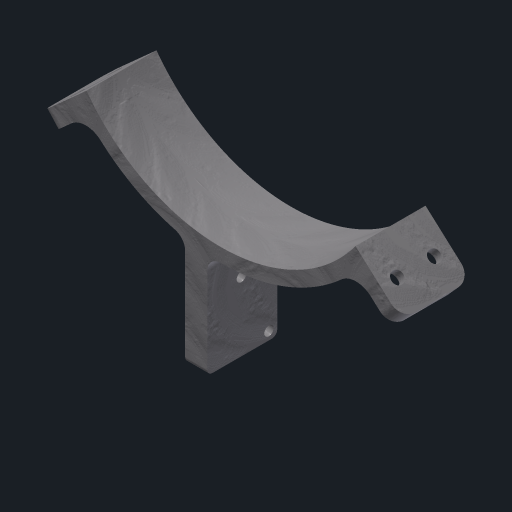
# Autodesk Inventor part: CANALETA_MOVIL
Saved by Autodesk Inventor 2024.3 (Build 283343000, 343)
## iProperties
Created: 2024-07-24
Part Number: CANALETA_MOVIL
Material: Steel, Mild, Welded
Document SubType Name: Modeling
Designer: Niler
Density: 7.85 g/cm^3
Appearance: Weld - Steel Mild
Author: Niler
Autodesk Inventor part; units mm, degrees
ref_plane "YZ Plane" through (0, 0, 0) normal (1, 0, 0) x (0, 1, 0)
ref_plane "XZ Plane" through (0, 0, 0) normal (0, 1, 0) x (-1, 0, 0)
ref_plane "XY Plane" through (0, 0, 0) normal (0, 0, 1) x (1, 0, 0)
sketch "Sketch1" plane through (0, 0, 0) normal (0, 0, 1) x (1, 0, 0)
  circle A0 centre (0, 0) radius 57.5
  circle A1 centre (0, 0) radius 60.5
  line L0 (0, 0) -> (-45, -40.4382)
  line L1 (0, 0) -> (0, 20.5864)
  line L2 (0, 0) -> (45, -40.4382)
  circle A2 centre (0, 0) radius 65.5
  line L3 (-45, -40.4382) -> (-48.719, -43.7802)
  line L4 (45, -40.4382) -> (48.719, -43.7802)
  line L5 (-4.7542, 3.7944) -> (-49.0104, -35.9754)
  line L6 (-49.0104, -35.9754) -> (-65.4381, -50.7378)
  line L7 (-48.719, -43.7802) -> (-61.4277, -55.2006)
  line L8 (-65.4381, -50.7378) -> (-61.4277, -55.2006)
  arc A3 (-43.6644, -48.8229) -> (-54.3446, -48.8356) centre (-48.9974, -54.786) ccw
  line L9 (49.0104, -35.9754) -> (65.4381, -50.7378)
  line L10 (48.719, -43.7802) -> (61.4277, -55.2006)
  line L11 (65.4381, -50.7378) -> (61.4277, -55.2006)
  arc A4 (54.3446, -48.8356) -> (43.6644, -48.8229) centre (48.9974, -54.786) ccw
  line L12 (4.7542, 3.7944) -> (49.0104, -35.9754)
  point P0 (45, -40.4382)
  point P1 (42.7686, -38.433)
  point P2 (-42.7686, -38.433)
  point P3 (-46.5455, -33.7604)
  point P4 (52.5246, -39.1333)
  point P5 (43.6644, -48.8229)
  point P6 (-48.7886, -35.7761)
  point P7 (48.7886, -35.7761)
  dimension "d0" = 115
  dimension "d1" = 3
  dimension "d2" = 90
  dimension "d5" = 5
  dimension "d6" = 6
  dimension "d7" = 25.4
  dimension "d8" = 8
  constraints: 28 end point, 8 symmetric about line, 7 point on circle, 4 collinear, 3 centre point, 3 point on line, 2 tangent, 1 coincident, 1 perpendicular, 1 vertical, 8 other
  measures "d2" distance of L2.end L0.end
  measures "d6" distance between parallel lines of L0 L5
  measures "d7" distance of L6.end point (-46.546, -33.76)
  measures "d8" radius of A3
extrude "Extrusion1" add sketch "Sketch1" along normal mid plane 25.4 contours A1 L3 A2 L6 L5 | L12 L9 A2 L4 A1 | A1 L4 A2 L3 | L7 L8 L6 A2 | A2 A3 L7 | L10 A4 A2 | A2 L9 L11 L10
fillet "Fillet1" radius 5 4 edges at (-63.4329, -52.9692, 12.7) (-63.4329, -52.9692, -12.7) (63.4329, -52.9692, 12.7) (63.4329, -52.9692, -12.7)
sketch "Sketch2" plane through (-54.3446, -48.8356, -12.7) normal (0.6684004, -0.7438017, 0) x (0.7438017, 0.6684004, 0)
  arc A0 (-9.5228, 5) -> (-4.5228, 0) centre (-4.5228, 5) ccw projected
  line L0 (0, 0) -> (-4.5228, 0) projected
  line L1 (0, 0) -> (0, 25.4) projected
  line L2 (-4.5228, 25.4) -> (0, 25.4) projected
  arc A1 (-4.5228, 25.4) -> (-9.5228, 20.4) centre (-4.5228, 20.4) ccw projected
  line L3 (-9.5228, 5) -> (-9.5228, 20.4) projected
  line L4 (7.9525, 0) -> (7.9525, 25.4) projected
  line L5 (0, 25.4) -> (7.9525, 25.4) projected
  line L6 (0, 0) -> (0, 25.4) projected
  line L7 (7.9525, 0) -> (0, 0) projected
  circle A2 centre (0.4772, 19.4) radius 2.15
  line L8 (-9.5228, 12.7) -> (-3.8871, 12.7)
  circle A3 centre (0.4772, 6) radius 2.15
  point P0 (73.0633, 12.7)
  point P1 (0, 21.4964)
  point P2 (0, 17.3036)
  dimension "d10" = 4.3
  dimension "d11" = 10
  dimension "d17" = 6
  constraints: 2 centre point, 2 end point, 1 horizontal, 1 midpoint, 1 symmetric about line, 1 other
  measures "d10" diameter of A2
  measures "d11" distance from line of L3 A2.centre
  measures "d17" distance from line of L2 A2.centre
extrude "Extrusion2" cut sketch "Sketch2" along normal through all both and the other way through all contours A3 L1 | L1 A3 | A2 L1 | L1 A2
sketch "Sketch3" plane through (-61.4277, -55.2006, -7.7) normal (0.6684004, -0.7438017, 0) x (0.7438017, 0.6684004, 0)
  arc A0 (9.5228, 16.4964) -> (9.5228, 12.3036) centre (10, 14.4) ccw projected
  line L0 (9.5228, 16.4964) -> (9.5228, 20.4) projected
  line L1 (5, 20.4) -> (9.5228, 20.4) projected
  arc A1 (5, 20.4) -> (0, 15.4) centre (5, 15.4) ccw projected
  line L2 (0, 0) -> (0, 15.4) projected
  arc A2 (0, 0) -> (5, -5) centre (5, 0) ccw projected
  line L3 (9.5228, -5) -> (5, -5) projected
  line L4 (9.5228, -5) -> (9.5228, -1.0964) projected
  circle A3 centre (10, 14.4) radius 4
  arc A4 (9.5228, 3.0964) -> (9.5228, -1.0964) centre (10, 1) ccw projected
  line L5 (9.5228, 3.0964) -> (9.5228, 12.3036) projected
  circle A5 centre (10, 1) radius 4
  point P0 (82.5861, 7.7)
  dimension "d14" = 8
  constraints: 2 centre point, 2 coincident, 1 equal radius
  measures "d14" diameter of A3
extrude "Extrusion3" cut sketch "Sketch3" along normal mid plane 6 contours L0 A3 L5 A0 | A0 L5 A3 L0 | A5 L4 A4 L5 | L5 A4 L4 A5
mirror "Mirror2" about plane through (0, 0, 0) normal (1, 0, 0) of "Extrusion3", "Extrusion2"
sketch "Sketch4" plane through (0, 0, -12.7) normal (0, 0, -1) x (-1, 0, 0)
  line L0 (-5, -65.5) -> (5, -65.5)
  line L1 (5, -65.5) -> (5, -103.5)
  line L2 (5, -103.5) -> (-5, -103.5)
  line L3 (-5, -103.5) -> (-5, -65.5)
  line L4 (-57.7087, -51.8586) -> (-61.7191, -47.3958) projected
  line L5 (-57.7087, -51.8586) -> (-54.3446, -48.8356) projected
  arc A0 (-43.6644, -48.8229) -> (-54.3446, -48.8356) centre (-48.9974, -54.786) ccw projected
  arc A1 (-43.6644, -48.8229) -> (43.6644, -48.8229) centre (0, 0) ccw projected
  arc A2 (54.3446, -48.8356) -> (43.6644, -48.8229) centre (48.9974, -54.786) ccw projected
  line L6 (54.3446, -48.8356) -> (57.7087, -51.8586) projected
  line L7 (61.7191, -47.3958) -> (57.7087, -51.8586) projected
  line L8 (61.7191, -47.3958) -> (48.7886, -35.7761) projected
  arc A3 (-48.7886, -35.7761) -> (48.7886, -35.7761) centre (0, 0) ccw projected
  line L9 (-48.7886, -35.7761) -> (-61.7191, -47.3958) projected
  line L10 (-5, -65.5) -> (5, -65.5)
  line L11 (5, -65.5) -> (5, -61.5)
  line L12 (5, -61.5) -> (-5, -61.5)
  line L13 (-5, -61.5) -> (-5, -65.5)
  line L14 (5, -61.5) -> (13, -61.5)
  line L15 (13, -61.5) -> (13, -103.5)
  line L16 (13, -103.5) -> (5, -103.5)
  line L17 (5, -103.5) -> (5, -61.5)
  point P0 (0, -65.5)
  point P1 (13, -64.197)
  point P2 (5, -65.3089)
  dimension "d18" = 10
  dimension "d19" = 38
  dimension "d20" = 4
  dimension "d21" = 8
  constraints: 24 end point, 6 parallel, 3 horizontal, 3 perpendicular, 1 midpoint, 1 point on circle
  measures "d18" distance between parallel lines of L1 L3
  measures "d19" distance of L2.end L0.start
  measures "d20" distance between parallel lines of L0 L12
  measures "d21" distance of L15.end L1.end
extrude "Extrusion4" add sketch "Sketch4" against normal up to surface (25.4 mm away) contours L11 A1 L15 L16 L1
sketch "Sketch5" plane through (-13, -103.5, -12.7) normal (-1, 0, 0) x (0, 0, 1)
  line L0 (25.4, 0) -> (25.4, 39.303) projected
  line L1 (0, 39.303) -> (25.4, 39.303) projected
  line L2 (0, 0) -> (0, 39.303) projected
  line L3 (0, 0) -> (25.4, 0) projected
  line L4 (0, 0) -> (16, 0)
  line L5 (16, 0) -> (16, 28)
  line L6 (16, 28) -> (0, 28)
  line L7 (0, 28) -> (0, 0)
  circle A0 centre (13, 25) radius 1.7
  circle A1 centre (3, 3) radius 1.7
  point P0 (12.7, 103.5)
  dimension "d24" = 16
  dimension "d25" = 28
  dimension "d26" = 3
  dimension "d27" = 3
  dimension "d28" = 3
  dimension "d29" = 3
  dimension "d30" = 3.4
  constraints: 8 end point, 2 centre point, 2 parallel, 1 equal radius, 1 horizontal, 1 perpendicular
  measures "d24" distance of L6.end L5.end
  measures "d25" distance of L5.end L4.end
  measures "d26" distance from line of L2 A1.centre
  measures "d27" distance from line of L3 A1.centre
  measures "d28" distance from line of L6 A0.centre
  measures "d29" distance from line of L5 A0.centre
  measures "d30" diameter of A1
extrude "Extrusion5" cut sketch "Sketch5" against normal through all contours A0 | A1
fillet "Fillet2" radius 2 2 edges at (-9, -103.5, -12.7) (-9, -103.5, 12.7)
fillet "Fillet3" radius 5 2 edges at (-13, -64.197, 0) (-5, -65.3089, 0)
body "Solid1"
